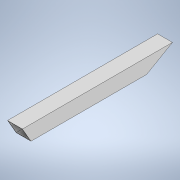
# Autodesk Inventor part: Деталь3
Saved by Autodesk Inventor 2022 (Build 260153000, 153)
## iProperties
Created: 2023-02-20
Part Number: Деталь3
Material: Типовые
Document SubType Name: Modeling
Designer: 89778080384
Density: 1 g/cm^3
Appearance: По умолчанию
Author: 89778080384
Autodesk Inventor part; units mm, degrees
ref_plane "YZ Plane" through (0, 0, 0) normal (1, 0, 0) x (0, 1, 0)
ref_plane "XZ Plane" through (0, 0, 0) normal (0, 1, 0) x (-1, 0, 0)
ref_plane "XY Plane" through (0, 0, 0) normal (0, 0, 1) x (1, 0, 0)
sketch "Эскиз1" plane through (0, 0, 0) normal (0, 0, 1) x (1, 0, 0)
  line L0 (10, -10) -> (-10, -10)
  line L1 (-10, -10) -> (-10, 10)
  line L2 (-10, 10) -> (10, 10)
  line L3 (10, 10) -> (10, -10)
  line L4 (10, -10) -> (-10, 10) construction
  line L5 (-10, -10) -> (10, 10) construction
  line L6 (9.25, -9.25) -> (-9.25, -9.25)
  line L7 (-9.25, -9.25) -> (-9.25, 9.25)
  line L8 (-9.25, 9.25) -> (9.25, 9.25)
  line L9 (9.25, 9.25) -> (9.25, -9.25)
  line L10 (9.25, -9.25) -> (-9.25, 9.25) construction
  line L11 (-9.25, -9.25) -> (9.25, 9.25) construction
  point P0 (0, 0)
  dimension "d0" = 20
  dimension "d1" = 20
  dimension "d2" = 18.5
  dimension "d3" = 18.5
  constraints: 24 end point, 4 midpoint, 4 parallel, 2 horizontal, 2 perpendicular
  measures "d0" distance of L1.end L2.end
  measures "d1" distance of L0.end L1.end
  measures "d2" distance of L7.end L8.end
  measures "d3" distance of L6.end L7.end
extrude "Выдавливание1" add sketch "Эскиз1" along normal blind 202.0726
sketch "Эскиз2" plane through (10, -10, 0) normal (1, 0, 0) x (0, 0, -1)
  line L0 (0, 0) -> (0, 20) projected
  line L1 (0, 20) -> (-34.641, 0)
  line L2 (0, 0) -> (-202.0726, 0) projected
  line L3 (0, 20) -> (40, 20) construction
  line L4 (-34.641, 0) -> (0, 0)
  line L5 (0, 0) -> (0, 20)
  point P0 (0, 10)
  dimension "d6" = 150
  constraints: 8 end point, 2 horizontal, 1 collinear, 1 equal length, 1 point on line
  measures "d6" angle of L1 L3
extrude "Выдавливание2" cut sketch "Эскиз2" against normal blind 178.9786
sketch "Эскиз3" plane through (10, -10, 202.0726) normal (1, 0, 0) x (0, 0, -1)
  line L0 (0, 20) -> (11.547, 0)
  line L1 (167.4316, 0) -> (0, 0) projected
  line L2 (0, 20) -> (23.094, 20) construction
  line L3 (11.547, 0) -> (0, 0)
  line L4 (0, 0) -> (0, 20) projected
  line L5 (0, 0) -> (0, 20)
  point P0 (202.0726, 10)
  dimension "d9" = 60
  constraints: 8 end point, 2 collinear, 1 equal length, 1 horizontal, 1 point on line
  measures "d9" angle of L0 L2
extrude "Выдавливание3" cut sketch "Эскиз3" against normal blind 202.0726
